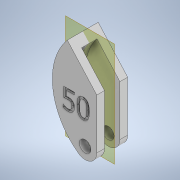
# Autodesk Inventor part: 05-1
Saved by Autodesk Inventor 2022 (Build 260153000, 153)
## iProperties
Created: 2021-09-11
Part Number: 05-1
Material: 일반
Document SubType Name: Modeling
Designer: 서울공업고등학교
Density: 1 g/cm^3
Appearance: 기본값
Mass: 7.17296 g
Surface Area: 45.3589 cm^2
Volume: 7.17296 cm^3
Author: 서울공업고등학교
Autodesk Inventor part; units mm, degrees
ref_plane "YZ Plane" through (0, 0, 0) normal (1, 0, 0) x (0, 1, 0)
ref_plane "XZ Plane" through (0, 0, 0) normal (0, 1, 0) x (-1, 0, 0)
sketch "스케치1" plane through (0, 0, 0) normal (0, 0, 1) x (1, 0, 0)
  line L0 (0, 0) -> (0, -26)
  line L1 (0, 0) -> (26, 0) construction
  arc A0 (-9.5556, -30.833) -> (0, -26) centre (-6, -26) ccw
  line L2 (0, 0) -> (-15.2463, 17)
  arc A1 (-15.2463, 17) -> (-9.5556, -30.833) centre (10, -4.2514) ccw
  circle A2 centre (-6, -26) radius 3
  dimension "d1" = 26
  dimension "d3" = 26
  dimension "d5" = 43
  dimension "d6" = 23
  dimension "d7" = 33
  dimension "d8" = 6
  dimension "d9" = 6
  constraints: 6 end point, 4 point on circle, 3 centre point, 1 coincident, 1 horizontal, 1 perpendicular, 1 tangent, 1 vertical
  measures "d1" distance of L0.start L0.end
  measures "d3" vertical distance of L0.start A0.centre
  measures "d5" vertical distance of A0.centre L2.end
  measures "d6" distance edge to line of A1 L0
  measures "d7" radius of A1
  measures "d8" radius of A0
  measures "d9" diameter of A2
extrude "돌출1" add sketch "스케치1" along normal mid plane 16
ref_plane "작업 평면1" through (0, 0, 0) normal (0, 0, -1) x (-1, 0, 0)
sketch "스케치2" plane through (0, 0, 0) normal (0, 0, -1) x (-1, 0, 0)
  arc A0 (9.5556, -30.833) -> (15.2463, 17) centre (-10, -4.2514) ccw projected
  line L0 (22.8853, -7) -> (17.8648, -7)
  line L1 (0, 0) -> (0, -26) projected
  circle A1 centre (6, -26) radius 3 projected
  arc A2 (17.8648, -7) -> (11.869, 13.2342) centre (-10, -4.2514) ccw
  line L2 (15.2463, 17) -> (0, 0) projected
  arc A3 (0, -26) -> (9.5556, -30.833) centre (6, -26) ccw projected
  dimension "d14" = 19
  constraints: 3 point on circle, 2 end point, 1 centre point, 1 horizontal, 1 point on line
  measures "d14" distance from line of L0 A1.centre
extrude "돌출2" cut sketch "스케치2" along normal mid plane 8 contours A3 L1 L2 A2 L0 A0
sketch "스케치6" plane through (0, 0, 8) normal (0, 0, 1) x (1, 0, 0)
  line L0 (-18.2733, -4.3259) -> (-3.2652, -4.3259) construction
  line L1 (-3.2652, -4.3259) -> (-3.2652, -14.7392) construction
  line L2 (-3.2652, -14.7392) -> (-18.2733, -14.7392) construction
  line L3 (-18.2733, -14.7392) -> (-18.2733, -4.3259) construction
  spline S0 degree 2 poles (-11.4824, -11.3519) (-11.4824, -12.0731) (-11.9443, -13.3049) (-12.3657, -13.7587) knots 0 0 0 1 2 2 2
  spline S1 degree 2 poles (-12.3657, -13.7587) (-12.7871, -14.2125) (-14.0432, -14.7392) (-14.8212, -14.7392) knots 0 0 0 1 2 2 2
  spline S2 degree 2 poles (-14.8212, -14.7392) (-15.5343, -14.7392) (-16.9281, -14.4232) (-17.4387, -14.172) knots 0 0 0 1 2 2 2
  line L4 (-17.4387, -14.172) -> (-17.4387, -12.7538)
  line L5 (-17.4387, -12.7538) -> (-17.3414, -12.7538)
  spline S3 degree 2 poles (-17.3414, -12.7538) (-17.1874, -12.8673) (-16.6121, -13.159) (-16.2636, -13.2887) knots 0 0 0 1 2 2 2
  spline S4 degree 2 poles (-16.2636, -13.2887) (-15.8665, -13.4264) (-15.2101, -13.5804) (-14.7968, -13.5804) knots 0 0 0 1 2 2 2
  spline S5 degree 2 poles (-14.7968, -13.5804) (-14.3917, -13.5804) (-13.6299, -13.2887) (-13.3544, -12.9726) knots 0 0 0 1 2 2 2
  spline S6 degree 2 poles (-13.3544, -12.9726) (-13.1032, -12.6728) (-12.8439, -11.8786) (-12.8439, -11.3438) knots 0 0 0 1 2 2 2
  spline S7 degree 2 poles (-12.8439, -11.3438) (-12.8439, -10.8089) (-13.1356, -10.1282) (-13.4111, -9.9013) knots 0 0 0 1 2 2 2
  spline S8 degree 2 poles (-13.4111, -9.9013) (-13.6947, -9.6501) (-14.5375, -9.4394) (-15.0481, -9.4394) knots 0 0 0 1 2 2 2
  spline S9 degree 2 poles (-15.0481, -9.4394) (-15.5991, -9.4394) (-16.6931, -9.6096) (-17.0254, -9.6825) knots 0 0 0 1 2 2 2
  line L6 (-17.0254, -9.6825) -> (-17.0254, -4.5285)
  line L7 (-17.0254, -4.5285) -> (-11.5392, -4.5285)
  line L8 (-11.5392, -4.5285) -> (-11.5392, -5.7036)
  line L9 (-11.5392, -5.7036) -> (-15.7369, -5.7036)
  line L10 (-15.7369, -5.7036) -> (-15.7369, -8.3697)
  spline S10 degree 2 poles (-15.7369, -8.3697) (-15.4938, -8.3373) (-15.0238, -8.313) (-14.8293, -8.313) knots 0 0 0 1 2 2 2
  spline S11 degree 2 poles (-14.8293, -8.313) (-14.0594, -8.313) (-12.9978, -8.5642) (-12.5116, -8.937) knots 0 0 0 1 2 2 2
  spline S12 degree 2 poles (-12.5116, -8.937) (-12.0173, -9.3097) (-11.4824, -10.4442) (-11.4824, -11.3519) knots 0 0 0 1 2 2 2
  spline S13 degree 2 poles (-3.8163, -9.5285) (-3.8163, -12.219) (-5.3803, -14.7392) (-7.0092, -14.7392) knots 0 0 0 1 2 2 2
  spline S14 degree 2 poles (-7.0092, -14.7392) (-8.6623, -14.7392) (-10.2101, -12.1703) (-10.2101, -9.5366) knots 0 0 0 1 2 2 2
  spline S15 degree 2 poles (-10.2101, -9.5366) (-10.2101, -6.83) (-8.6461, -4.3259) (-7.0092, -4.3259) knots 0 0 0 1 2 2 2
  spline S16 degree 2 poles (-7.0092, -4.3259) (-5.3641, -4.3259) (-3.8163, -6.9191) (-3.8163, -9.5285) knots 0 0 0 1 2 2 2
  spline S17 degree 2 poles (-5.5343, -12.5755) (-5.3398, -12.0812) (-5.1777, -10.5577) (-5.1777, -9.5285) knots 0 0 0 1 2 2 2
  spline S18 degree 2 poles (-5.1777, -9.5285) (-5.1777, -8.4994) (-5.3398, -6.984) (-5.5424, -6.4734) knots 0 0 0 1 2 2 2
  spline S19 degree 2 poles (-5.5424, -6.4734) (-5.745, -5.9629) (-6.45, -5.4361) (-7.0092, -5.4361) knots 0 0 0 1 2 2 2
  spline S20 degree 2 poles (-7.0092, -5.4361) (-7.5683, -5.4361) (-8.2896, -5.9629) (-8.5003, -6.4896) knots 0 0 0 1 2 2 2
  spline S21 degree 2 poles (-8.5003, -6.4896) (-8.7028, -7.0002) (-8.8487, -8.5561) (-8.8487, -9.5366) knots 0 0 0 1 2 2 2
  spline S22 degree 2 poles (-8.8487, -9.5366) (-8.8487, -10.5901) (-8.7191, -12.0002) (-8.5084, -12.5512) knots 0 0 0 1 2 2 2
  spline S23 degree 2 poles (-8.5084, -12.5512) (-8.3139, -13.0699) (-7.5926, -13.629) (-7.0092, -13.629) knots 0 0 0 1 2 2 2
  spline S24 degree 2 poles (-7.0092, -13.629) (-6.4581, -13.629) (-5.7369, -13.1023) (-5.5343, -12.5755) knots 0 0 0 1 2 2 2
  point P0 (0, 0)
  constraints: 2 other
extrude "돌출3" cut sketch "스케치6" against normal blind 1
